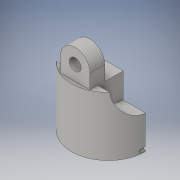
# Autodesk Inventor part: GERMI01-02-01
Saved by Autodesk Inventor 2016 (Build 200138000, 138)
## iProperties
Created: 2016-11-08
Part Number: GERMI01-02-01
Material: Generic
Document SubType Name: Modeling
Designer: Kai
Density: 1 g/cm^3
Appearance: Default
Author: Kai
Autodesk Inventor part; units mm, degrees
ref_plane "YZ Plane" through (0, 0, 0) normal (1, 0, 0) x (0, 1, 0)
ref_plane "XZ Plane" through (0, 0, 0) normal (0, 1, 0) x (-1, 0, 0)
ref_plane "XY Plane" through (0, 0, 0) normal (0, 0, 1) x (1, 0, 0)
sketch "Sketch1" plane through (0, 0, 0) normal (0, 1, 0) x (-1, 0, 0)
  arc A0 (15.875, 0) -> (-15.875, 0) centre (0, 0) ccw
  line L0 (15.875, 0) -> (-15.875, 0)
  dimension "d3" = 31.75
  constraints: 2 end point, 2 point on circle, 1 centre point, 1 horizontal
  measures "d3" diameter of A0
extrude "Extrusion1" add sketch "Sketch1" along normal blind 25.4
sketch "Sketch2" plane through (15.875, 0, 0) normal (0, 0, -1) x (-1, 0, 0)
  line L0 (19.685, 0) -> (19.685, 4.572)
  line L1 (19.685, 4.572) -> (21.463, 4.572)
  line L2 (21.463, 4.572) -> (21.463, 6.858)
  line L3 (15.875, 0) -> (15.875, 6.858)
  line L4 (21.463, 6.858) -> (15.875, 6.858)
  line L5 (19.685, 0) -> (15.875, 0)
  line L6 (31.75, 0) -> (0, 0) projected
  dimension "d12" = 1.778
  constraints: 12 end point, 2 horizontal, 1 collinear, 1 perpendicular, 1 vertical
  measures "d12" distance of L0.end L1.end
revolve "Revolution1" cut sketch "Sketch2" angle 360 about axis through (0, 0, 0) along (0, 1, 0)
sketch "Sketch3" plane through (0, 0, 0) normal (1, 0, 0) x (0, 1, 0)
  line L0 (25.4, 0) -> (25.4, 15.875) projected
  circle A0 centre (25.4, 0) radius 10.9033
  point P0 (0, 0)
  constraints: 1 centre point
extrude "Extrusion2" cut sketch "Sketch3" along normal mid plane 2540
sketch "Sketch4" plane through (0, 25.4, 0) normal (0, 1, 0) x (1, 0, 0)
  line L0 (13.7482, -7.9375) -> (-13.7482, -7.9375) projected
  line L1 (0, -7.9375) -> (-6.35, -7.9375)
  line L2 (-6.35, -7.9375) -> (-6.35, -14.2875)
  line L3 (-6.35, -14.2875) -> (6.35, -14.2875)
  line L4 (6.35, -14.2875) -> (6.35, -7.9375)
  line L5 (0, -7.9375) -> (6.35, -7.9375)
  line L6 (-6.35, -7.9375) -> (-6.35, 0)
  line L7 (-3.81, 0) -> (-15.875, 0) projected
  line L8 (-6.35, 0) -> (6.35, 0)
  line L9 (6.35, 0) -> (6.35, -7.9375)
  point P0 (0, 0)
  dimension "d17" = 6.35
  dimension "d18" = 6.35
  dimension "d19" = 12.7
  constraints: 16 end point, 4 perpendicular, 4 point on line, 1 horizontal, 1 midpoint, 1 vertical
  measures "d17" distance of L1.start L1.end
  measures "d18" distance of L1.end L2.end
  measures "d19" distance of L2.end L3.end
extrude "Extrusion3" add sketch "Sketch4" against normal blind 12.7 contours L0 L6 L7 L8 L9
extrude "Extrusion4" add sketch "Sketch4" along normal blind 2.54 contours L4 L3 L2 L0
sketch "Sketch7" plane through (6.35, 25.4, 7.9375) normal (0, 0, -1) x (-1, 0, 0)
  line L0 (12.7, 0) -> (12.7, 2.54) projected
  line L1 (0, 0) -> (12.7, 0) projected
  arc A0 (12.7, 6.35) -> (0, 6.35) centre (6.35, 6.35) ccw
  circle A1 centre (6.35, 6.35) radius 2.54
  line L2 (12.7, 6.35) -> (12.7, 2.54)
  line L3 (12.7, 2.54) -> (0, 2.54)
  line L4 (0, 2.54) -> (0, 6.35)
  point P0 (6.35, -25.4)
  dimension "d31" = 5.08
  constraints: 6 end point, 2 centre point, 2 point on circle, 1 coincident, 1 horizontal, 1 perpendicular, 1 vertical
  measures "d31" diameter of A1
extrude "Extrusion6" add sketch "Sketch7" against normal blind 6.35
ref_plane "Work Plane1" through (16.51, 17.4625, 0) normal (1, 0, 0) x (0, 0, -1)
sketch "Sketch10" plane through (16.51, 17.4625, 0) normal (1, 0, 0) x (0, 0, -1)
  arc A0 (-1.905, -15.5575) -> (-1.905, -16.8275) centre (-1.905, -16.1925) ccw
  line L0 (-1.905, -15.5575) -> (0, -15.5575)
  line L1 (0, -15.5575) -> (0, -16.8275)
  line L2 (-1.905, -16.8275) -> (0, -16.8275)
  circle A1 centre (-1.905, -16.1925) radius 0.635
  constraints: 6 end point, 2 centre point, 2 point on circle, 1 coincident, 1 concentric, 1 horizontal, 1 perpendicular, 1 tangent
extrude "Extrusion7" cut sketch "Sketch10" against normal blind 1.27
extrude "Extrusion8" cut sketch "Sketch10" against normal blind 2.54 contours A1 A0
mirror "Mirror1" about plane through (0, 0, 0) normal (1, 0, 0) of "Extrusion7", "Extrusion8"
sketch "Sketch14" plane through (15.875, 0, 0) normal (0, 0, -1) x (-1, 0, 0)
  line L0 (9.525, 14.4967) -> (9.525, 17.9248) projected
  line L1 (31.75, 14.4967) -> (22.225, 14.4967) projected
  line L2 (9.525, 14.4967) -> (22.225, 14.4967)
  line L3 (22.225, 25.4) -> (22.225, 17.9248) projected
  line L4 (22.225, 14.4967) -> (22.225, 25.4)
  line L5 (9.525, 25.4) -> (22.225, 25.4) projected
  line L6 (22.225, 25.4) -> (9.525, 25.4)
  line L7 (9.525, 25.4) -> (9.525, 14.4967)
  point P0 (15.875, 0)
  constraints: 8 end point, 2 collinear, 2 perpendicular
extrude "Extrusion9" add sketch "Sketch14" against normal blind 12.7
body "Solid1"
